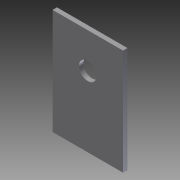
# Autodesk Inventor part: gearmotor mounting plate
Saved by Autodesk Inventor 2011 SP1 (Build 150282100, 282)
## iProperties
Created: 2012-01-20
Part Number: gearmotor mounting plate
Document SubType Name: Modeling
Designer: Christopher
Density: 1 g/cm^3
Author: Christopher
Autodesk Inventor part; units mm, degrees
ref_plane "YZ Plane" through (0, 0, 0) normal (1, 0, 0) x (0, 1, 0)
ref_plane "XZ Plane" through (0, 0, 0) normal (0, 1, 0) x (-1, 0, 0)
ref_plane "XY Plane" through (0, 0, 0) normal (0, 0, 1) x (1, 0, 0)
sketch "Sketch1" plane through (0, 0, 0) normal (0, 0, 1) x (1, 0, 0)
  line L0 (0, 0) -> (0, 79.375)
  line L1 (0, 79.375) -> (-50.8, 79.375)
  line L2 (-50.8, 79.375) -> (-50.8, 25.4)
  line L3 (-50.8, 25.4) -> (-50.8, 0)
  line L4 (-50.8, 0) -> (0, 0)
  circle A0 centre (-25.4, 53.975) radius 6.35
  dimension "d0" = 79.375
  dimension "d1" = 50.8
  dimension "d2" = 25.4
  dimension "d3" = 50.8
  dimension "d4" = 25.4
  dimension "d5" = 25.4
  dimension "d6" = 12.7
  constraints: 10 end point, 2 parallel, 1 centre point, 1 coincident, 1 perpendicular, 1 vertical
  measures "d0" distance of L0.start L0.end
  measures "d1" distance of L3.end L0.start
  measures "d2" distance of L2.end L3.end
  measures "d3" distance of L0.end L1.end
  measures "d4" distance from line of L0 point (-25.4, 53.975)
  measures "d5" distance from line of L1 point (-25.4, 53.975)
  measures "d6" diameter of A0
extrude "Extrusion1" add sketch "Sketch1" against normal blind 3.175
body "Solid1"
